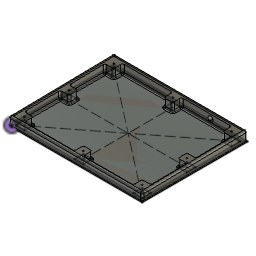
case (Autodesk Fusion 360 design; units mm, degrees)
Autodesk Fusion 360 part; units mm, degrees
sketch "Sketch1" plane through (0, 0, 0) normal (0, 0, 1) x (1, 0, 0)
  line L0 (0, 0) -> (294.692, 0)
  line L1 (294.692, 0) -> (294.692, 230.4)
  line L2 (294.692, 230.4) -> (0, 230.4)
  line L3 (0, 230.4) -> (0, 0)
  line L4 (-4, 234.4) -> (298.692, 234.4)
  line L5 (298.692, 234.4) -> (298.692, -4)
  line L6 (298.692, -4) -> (-4, -4)
  line L7 (-4, -4) -> (-4, 234.4)
  line L8 (4, 226.4) -> (290.692, 226.4)
  line L9 (290.692, 226.4) -> (290.692, 4)
  line L10 (290.692, 4) -> (4, 4)
  line L11 (4, 4) -> (4, 226.4)
  line L12 (4, 226.4) -> (24, 226.4)
  line L13 (24, 226.4) -> (24, 206.4)
  line L14 (24, 206.4) -> (4, 206.4)
  line L15 (4, 206.4) -> (4, 226.4)
  line L16 (4, 4) -> (24, 4)
  line L17 (24, 4) -> (24, 24)
  line L18 (24, 24) -> (4, 24)
  line L19 (4, 24) -> (4, 4)
  line L20 (290.692, 226.4) -> (270.692, 226.4)
  line L21 (270.692, 226.4) -> (270.692, 206.4)
  line L22 (270.692, 206.4) -> (290.692, 206.4)
  line L23 (290.692, 206.4) -> (290.692, 226.4)
  line L24 (290.692, 4) -> (270.692, 4)
  line L25 (270.692, 4) -> (270.692, 24)
  line L26 (270.692, 24) -> (290.692, 24)
  line L27 (290.692, 24) -> (290.692, 4)
  line L28 (4, 4) -> (290.692, 226.4) construction
  line L29 (4, 226.4) -> (290.692, 4) construction
  line L30 (147.346, 4) -> (147.346, 226.4) construction
  line L31 (290.692, 115.2) -> (4, 115.2) construction
  line L32 (137.346, 226.4) -> (157.346, 226.4)
  line L33 (157.346, 226.4) -> (157.346, 206.4)
  line L34 (157.346, 206.4) -> (137.346, 206.4)
  line L35 (137.346, 206.4) -> (137.346, 226.4)
  line L36 (137.346, 4) -> (157.346, 4)
  line L37 (157.346, 4) -> (157.346, 24)
  line L38 (157.346, 24) -> (137.346, 24)
  line L39 (137.346, 24) -> (137.346, 4)
  line L40 (4, 125.2) -> (24, 125.2)
  line L41 (24, 125.2) -> (24, 105.2)
  line L42 (24, 105.2) -> (4, 105.2)
  line L43 (4, 105.2) -> (4, 125.2)
  line L44 (290.692, 125.2) -> (270.692, 125.2)
  line L45 (270.692, 125.2) -> (270.692, 105.2)
  line L46 (270.692, 105.2) -> (290.692, 105.2)
  line L47 (290.692, 105.2) -> (290.692, 125.2)
  line L48 (4, 206.4) -> (24, 226.4) construction
  line L49 (4, 226.4) -> (24, 206.4) construction
  line L50 (137.346, 226.4) -> (157.346, 206.4) construction
  line L51 (137.346, 206.4) -> (157.346, 226.4) construction
  line L52 (4, 125.2) -> (24, 105.2) construction
  line L53 (4, 105.2) -> (24, 125.2) construction
  line L54 (24, 24) -> (4, 4) construction
  line L55 (4, 24) -> (24, 4) construction
  line L56 (137.346, 24) -> (157.346, 4) construction
  line L57 (137.346, 4) -> (157.346, 24) construction
  line L58 (270.692, 24) -> (290.692, 4) construction
  line L59 (270.692, 4) -> (290.692, 24) construction
  line L60 (270.692, 105.2) -> (290.692, 125.2) construction
  line L61 (270.692, 125.2) -> (290.692, 105.2) construction
  line L62 (270.692, 206.4) -> (290.692, 226.4) construction
  line L63 (270.692, 226.4) -> (290.692, 206.4) construction
  dimension "d1" = 294.692
  dimension "d2" = 230.4
  dimension "d3" = 4
  dimension "d4" = 4
  dimension "d5" = 4
  dimension "d6" = 4
  dimension "d7" = 4
  dimension "d8" = 4
  dimension "d9" = 4
  dimension "d10" = 4
  dimension "d11" = 20
  dimension "d12" = 20
  dimension "d13" = 20
  dimension "d14" = 20
  dimension "d15" = 20
  dimension "d16" = 20
  dimension "d17" = 20
  dimension "d18" = 20
  dimension "d19" = 20
  dimension "d20" = 20
  dimension "d21" = 20
  dimension "d22" = 20
  dimension "d23" = 20
  dimension "d24" = 20
  dimension "d25" = 20
  dimension "d26" = 20
  constraint horizontal L0
  constraint vertical L1
  constraint horizontal L2
  constraint vertical L3
  constraint coincident L0.start L3.end
  constraint horizontal L4
  constraint vertical L5
  constraint horizontal L6
  constraint vertical L7
  constraint horizontal L8
  constraint vertical L9
  constraint horizontal L10
  constraint vertical L11
  constraint horizontal L12
  constraint vertical L13
  constraint horizontal L14
  constraint vertical L15
  constraint horizontal L16
  constraint vertical L17
  constraint horizontal L18
  constraint vertical L19
  constraint horizontal L20
  constraint vertical L21
  constraint horizontal L22
  constraint vertical L23
  constraint horizontal L24
  constraint vertical L25
  constraint horizontal L26
  constraint vertical L27
  constraint midpoint L10 L30.start
  constraint midpoint L8 L30.end
  constraint midpoint L9 L31.start
  constraint midpoint L11 L31.end
  constraint horizontal L32
  constraint vertical L33
  constraint horizontal L34
  constraint vertical L35
  constraint coincident L8 L32.start
  constraint symmetric L30 L33 L35
  constraint horizontal L36
  constraint vertical L37
  constraint horizontal L38
  constraint vertical L39
  constraint coincident L10 L36.start
  constraint symmetric L30 L37 L39
  constraint horizontal L40
  constraint vertical L41
  constraint horizontal L42
  constraint vertical L43
  constraint coincident L11 L40.start
  constraint symmetric L31 L40 L42
  constraint horizontal L44
  constraint vertical L45
  constraint horizontal L46
  constraint vertical L47
  constraint coincident L9 L44.start
  constraint symmetric L31 L44 L46
  measures "d1" distance of L0.start L0.end
  measures "d2" distance of L0.start L2.end
  measures "d3" distance of L3 L7
  measures "d4" distance of L2 L4
  measures "d5" distance of L1 L5
  measures "d6" distance of L0 L6
  measures "d7" distance of L3 L11
  measures "d8" distance of L2 L8
  measures "d9" distance of L0 L10
  measures "d10" distance of L1 L9
  measures "d11" distance of L8.start L12.end
  measures "d12" distance of L8.start L14.end
  measures "d13" distance of L10.end L16.end
  measures "d14" distance of L10.end L18.end
  measures "d15" distance of L8.end L20.end
  measures "d16" distance of L8.end L22.end
  measures "d17" distance of L9.end L24.end
  measures "d18" distance of L9.end L26.end
  measures "d19" distance of L32.start L32.end
  measures "d20" distance of L32.start L34.end
  measures "d21" distance of L36.start L36.end
  measures "d22" distance of L36.start L38.end
  measures "d23" distance of L40.start L40.end
  measures "d24" distance of L40.start L42.end
  measures "d25" distance of L44.start L44.end
  measures "d26" distance of L44.start L46.end
extrude "Extrude1" add sketch "Sketch1" along normal blind 20 contours L0 L1 L2 L3 | L4 L5 L6 L7 | L8 L11 L12 L13 L14 L15 | L8 L32 L33 L34 L35 | L11 L40 L41 L42 L43 | L8 L9 L20 L21 L22 L23 | L10 L11 L16 L17 L18 L19 | L9 L44 L45 L46 L47 | L10 L36 L37 L38 L39 | L9 L10 L24 L25 L26 L27
extrude "Extrude2" add sketch "Sketch1" against normal blind 2 contours L0 L1 L2 L3 | L4 L5 L6 L7 | L8 L11 L12 L13 L14 L15 | L8 L9 L10 L11 L13 L14 L17 L18 L21 L22 L25 L26 L33 L34 L35 L37 L38 L39 L40 L41 L42 L44 L45 L46 | L8 L32 L33 L34 L35 | L11 L40 L41 L42 L43 | L8 L9 L20 L21 L22 L23 | L10 L11 L16 L17 L18 L19 | L9 L44 L45 L46 L47 | L10 L36 L37 L38 L39 | L9 L10 L24 L25 L26 L27
fillet "Fillet1" radius 4 28 edges at (24, 226.4, 10) (24, 206.4, 10) (4, 206.4, 10) (4, 125.2, 10) (24, 125.2, 10) (24, 105.2, 10) (4, 105.2, 10) (4, 24, 10) (24, 24, 10) (24, 4, 10) (137.346, 4, 10) (137.346, 24, 10) (157.346, 24, 10) (157.346, 4, 10) (270.692, 4, 10) (270.692, 24, 10) (290.692, 24, 10) (137.346, 226.4, 10) (137.346, 206.4, 10) (157.346, 206.4, 10) (157.346, 226.4, 10) (270.692, 226.4, 10) (270.692, 206.4, 10) (290.692, 206.4, 10) (290.692, 125.2, 10) (270.692, 125.2, 10) (270.692, 105.2, 10) (290.692, 105.2, 10)
fillet "Fillet2" radius 4 56 edges at (136.1744, 225.2284, 0) (80.673, 226.4, 0) (25.1716, 225.2284, 0) (24, 216.4, 0) (22.8284, 207.5716, 0) (14, 206.4, 0) (5.1716, 205.2284, 0) (4, 165.8, 0) (5.1716, 126.3716, 0) (14, 125.2, 0) (22.8284, 124.0284, 0) (24, 115.2, 0) (22.8284, 106.3716, 0) (14, 105.2, 0) (5.1716, 104.0284, 0) (4, 64.6, 0) (5.1716, 25.1716, 0) (14, 24, 0) (22.8284, 22.8284, 0) (24, 14, 0) (25.1716, 5.1716, 0) (80.673, 4, 0) (136.1744, 5.1716, 0) (137.346, 14, 0) (138.5176, 22.8284, 0) (147.346, 24, 0) (156.1744, 22.8284, 0) (157.346, 14, 0) (158.5176, 5.1716, 0) (214.019, 4, 0) (269.5204, 5.1716, 0) (270.692, 14, 0) (271.8636, 22.8284, 0) (280.692, 24, 0) (289.5204, 25.1716, 0) (290.692, 64.6, 0) (289.5204, 104.0284, 0) (280.692, 105.2, 0) (271.8636, 106.3716, 0) (270.692, 115.2, 0) (271.8636, 124.0284, 0) (280.692, 125.2, 0) (289.5204, 126.3716, 0) (290.692, 165.8, 0) (289.5204, 205.2284, 0) (280.692, 206.4, 0) (271.8636, 207.5716, 0) (270.692, 216.4, 0) (269.5204, 225.2284, 0) (214.019, 226.4, 0) (158.5176, 225.2284, 0) (157.346, 216.4, 0) (156.1744, 207.5716, 0) (147.346, 206.4, 0) (138.5176, 207.5716, 0) (137.346, 216.4, 0)
sketch "Sketch2" plane through (0, 0, 20) normal (0, 0, 1) x (-1, 0, 0)
  arc A0 (-270.692, -109.2) -> (-274.692, -105.2) centre (-274.692, -109.2) ccw
  line L0 (-274.692, -105.2) -> (-286.692, -105.2)
  arc A1 (-290.692, -101.2) -> (-286.692, -105.2) centre (-286.692, -101.2) ccw
  line L1 (-290.692, -101.2) -> (-290.692, -28)
  arc A2 (-286.692, -24) -> (-290.692, -28) centre (-286.692, -28) ccw
  line L2 (-286.692, -24) -> (-274.692, -24)
  arc A3 (-274.692, -24) -> (-270.692, -20) centre (-274.692, -20) ccw
  line L3 (-270.692, -20) -> (-270.692, -8)
  arc A4 (-266.692, -4) -> (-270.692, -8) centre (-266.692, -8) ccw
  line L4 (-266.692, -4) -> (-161.346, -4)
  arc A5 (-157.346, -8) -> (-161.346, -4) centre (-161.346, -8) ccw
  line L5 (-157.346, -8) -> (-157.346, -20)
  arc A6 (-157.346, -20) -> (-153.346, -24) centre (-153.346, -20) ccw
  line L6 (-153.346, -24) -> (-141.346, -24)
  arc A7 (-141.346, -24) -> (-137.346, -20) centre (-141.346, -20) ccw
  line L7 (-137.346, -20) -> (-137.346, -8)
  arc A8 (-133.346, -4) -> (-137.346, -8) centre (-133.346, -8) ccw
  line L8 (-133.346, -4) -> (-28, -4)
  arc A9 (-24, -8) -> (-28, -4) centre (-28, -8) ccw
  line L9 (-24, -8) -> (-24, -20)
  arc A10 (-24, -20) -> (-20, -24) centre (-20, -20) ccw
  line L10 (-20, -24) -> (-8, -24)
  arc A11 (-4, -28) -> (-8, -24) centre (-8, -28) ccw
  line L11 (-4, -28) -> (-4, -101.2)
  arc A12 (-8, -105.2) -> (-4, -101.2) centre (-8, -101.2) ccw
  line L12 (-8, -105.2) -> (-20, -105.2)
  arc A13 (-20, -105.2) -> (-24, -109.2) centre (-20, -109.2) ccw
  line L13 (-24, -109.2) -> (-24, -121.2)
  arc A14 (-24, -121.2) -> (-20, -125.2) centre (-20, -121.2) ccw
  line L14 (-20, -125.2) -> (-8, -125.2)
  arc A15 (-4, -129.2) -> (-8, -125.2) centre (-8, -129.2) ccw
  line L15 (-4, -129.2) -> (-4, -202.4)
  arc A16 (-8, -206.4) -> (-4, -202.4) centre (-8, -202.4) ccw
  line L16 (-8, -206.4) -> (-20, -206.4)
  arc A17 (-20, -206.4) -> (-24, -210.4) centre (-20, -210.4) ccw
  line L17 (-24, -210.4) -> (-24, -222.4)
  arc A18 (-28, -226.4) -> (-24, -222.4) centre (-28, -222.4) ccw
  line L18 (-28, -226.4) -> (-133.346, -226.4)
  arc A19 (-137.346, -222.4) -> (-133.346, -226.4) centre (-133.346, -222.4) ccw
  line L19 (-137.346, -222.4) -> (-137.346, -210.4)
  arc A20 (-137.346, -210.4) -> (-141.346, -206.4) centre (-141.346, -210.4) ccw
  line L20 (-141.346, -206.4) -> (-153.346, -206.4)
  arc A21 (-153.346, -206.4) -> (-157.346, -210.4) centre (-153.346, -210.4) ccw
  line L21 (-157.346, -210.4) -> (-157.346, -222.4)
  arc A22 (-161.346, -226.4) -> (-157.346, -222.4) centre (-161.346, -222.4) ccw
  line L22 (-161.346, -226.4) -> (-266.692, -226.4)
  arc A23 (-270.692, -222.4) -> (-266.692, -226.4) centre (-266.692, -222.4) ccw
  line L23 (-270.692, -222.4) -> (-270.692, -210.4)
  arc A24 (-270.692, -210.4) -> (-274.692, -206.4) centre (-274.692, -210.4) ccw
  line L24 (-274.692, -206.4) -> (-286.692, -206.4)
  arc A25 (-290.692, -202.4) -> (-286.692, -206.4) centre (-286.692, -202.4) ccw
  line L25 (-290.692, -202.4) -> (-290.692, -129.2)
  arc A26 (-286.692, -125.2) -> (-290.692, -129.2) centre (-286.692, -129.2) ccw
  line L26 (-286.692, -125.2) -> (-274.692, -125.2)
  arc A27 (-274.692, -125.2) -> (-270.692, -121.2) centre (-274.692, -121.2) ccw
  line L27 (-270.692, -121.2) -> (-270.692, -109.2)
  line L28 (4, 4) -> (-298.692, 4)
  line L29 (-298.692, 4) -> (-298.692, -234.4)
  line L30 (-298.692, -234.4) -> (4, -234.4)
  line L31 (4, -234.4) -> (4, 4)
  line L32 (0, -230.4) -> (-294.692, -230.4)
  line L33 (-294.692, -230.4) -> (-294.692, 0)
  line L34 (-294.692, 0) -> (0, 0)
  line L35 (0, 0) -> (0, -230.4)
  dimension "d35" = 4
  dimension "d36" = 4
  dimension "d37" = 4
  dimension "d38" = 4
  constraint horizontal L32
  constraint vertical L33
  constraint horizontal L34
  constraint vertical L35
  measures "d35" distance of L31 L35
  measures "d36" distance of L30 L32
  measures "d37" distance of L28 L34
  measures "d38" distance of L29 L33
sketch "Sketch3" plane through (-4, 0, 0) normal (-1, 0, 0) x (0, -1, 0)
  line L0 (4, -2) -> (4, 20)
  line L1 (4, 20) -> (-234.4, 20)
  line L2 (-234.4, 20) -> (-234.4, -2)
  line L3 (-234.4, -2) -> (4, -2)
  line L4 (4, -2) -> (4, 16)
  line L5 (4, 16) -> (-234.4, 20)
  dimension "d39" = 18
  constraint coincident L0.start L3.end
  constraint perpendicular L3 L4
  constraint coincident L1.end L2.start
  measures "d39" distance of L0.start L4.end
extrude "Extrude3" cut sketch "Sketch3" against normal through all contours L0 L1 L5
extrude "Extrude4" add sketch "Sketch2" against normal through all of body 1 contours L28 L29 L30 L31
extrude "Extrude5" add 1 faces at (196.4613, -2.6667, 20) along direction (0, 0, 1) blind 3
sketch "Sketch4" plane through (-4, 0, 0) normal (-1, 0, 0) x (0, -1, 0)
  line L0 (-234.4, 23) -> (-234.4, -2)
  line L1 (-234.4, -2) -> (4, -2)
  line L2 (4, -2) -> (4, 23)
  line L3 (4, 23) -> (-234.4, 23)
  line L4 (4, -2) -> (4, 19)
  line L5 (4, 19) -> (-234.4, 23)
  dimension "d44" = 21
  constraint coincident L1.end L2.start
  constraint perpendicular L1 L4
  constraint coincident L0.start L3.end
  measures "d44" distance of L1.end L4.end
extrude "Extrude6" cut sketch "Sketch4" against normal through all contours L2 L3 L5
sketch "Sketch5" plane through (0, 234.4, 0) normal (0, 1, 0) x (-1, 0, 0)
  line L0 (4, -2) -> (4, 23)
  line L1 (4, 23) -> (-298.692, 23)
  line L2 (-298.692, 23) -> (-298.692, -2)
  line L3 (-298.692, -2) -> (4, -2)
  line L4 (-298.692, -2) -> (4, 23) construction
  line L5 (4, -2) -> (-298.692, 23) construction
  line L6 (-147.346, 23) -> (-147.346, -2) construction
  line L7 (-298.692, -2) -> (-147.346, 23) construction
  line L8 (-147.346, -2) -> (-298.692, 23) construction
  circle A0 centre (-223.019, 10.5) radius 5.6
  line L9 (-225.0975, 15.7) -> (-220.9405, 15.7)
  line L10 (-225.0975, 5.3) -> (-220.9405, 5.3)
  dimension "d46" = 11.2
  dimension "d47" = 10.4
  constraint coincident L2.end L3.start
  constraint coincident L0.end L1.start
  constraint coincident L0.start L3.end
  constraint coincident L1.end L2.start
  constraint midpoint L1 L6.start
  constraint midpoint L3 L6.end
  constraint midpoint L7 A0.centre
  constraint coincident A0 L9.start
  constraint coincident A0 L9.end
  constraint horizontal L9
  constraint coincident A0 L10.start
  constraint coincident A0 L10.end
  constraint horizontal L10
  constraint equal L9 L10
  measures "d46" diameter of A0
  measures "d47" distance of L9 L10
extrude "Extrude7" cut sketch "Sketch5" against normal blind 8 contours A0 L9 L10
fillet "Fillet3" radius 2 4 edges at (0, 230.4, 21.4329) (0, 0, 17.5671) (294.692, 0, 17.5671) (294.692, 230.4, 21.4329)
fillet "Fillet4" radius 4 4 edges at (298.692, -4, 8.5) (298.692, 234.4, 10.5) (-4, -4, 8.5) (-4, 234.4, 10.5)
fillet "Fillet5" radius 4 16 edges at (-2.8284, -2.8284, -2) (-4, 115.2, -2) (-2.8284, 233.2284, -2) (147.346, 234.4, -2) (297.5204, 233.2284, -2) (298.692, 115.2, -2) (297.5204, -2.8284, -2) (147.346, -4, -2) (147.346, 234.4, 23) (297.5204, 233.2284, 22.9803) (298.692, 115.2, 21) (297.5204, -2.8284, 19.0197) (147.346, -4, 19) (-2.8284, -2.8284, 19.0197) (-4, 115.2, 21) (-2.8284, 233.2284, 22.9803)
hole "Hole1" at (14, 216.3986, 19.698) direction (0, 0.016776, -0.999859) diameter 3.332 depth 8 tip angle 118
thread "Thread1" "ISO Metric profile 4.0 M4x0.7 6H" major diameter 4.1095 minor diameter 3.332 pitch 0.7 angle 60 resizes the face on face at (12.6473, 215.4709, 17.0154)
hole "Hole2" at (147.346, 216.3986, 19.698) direction (0, 0.016776, -0.999859) diameter 3.332 depth 10 tip angle 118
thread "Thread2" "ISO Metric profile 4.0 M4x0.7 6H" thread offset 0 thread depth 7.4
hole "Hole3" at (280.692, 216.3986, 19.698) direction (0, 0.016776, -0.999859) diameter 3.332 depth 10 tip angle 118
thread "Thread3" "ISO Metric profile 4.0 M4x0.7 6H" thread offset 0 thread depth 7.4
hole "Hole4" at (280.692, 115.2014, 18) direction (0, 0.016776, -0.999859) diameter 3.332 depth 10 tip angle 118
thread "Thread4" "ISO Metric profile 4.0 M4x0.7 6H" thread offset 0 thread depth 7.4
hole "Hole5" at (280.692, 14.0014, 16.302) direction (0, 0.016776, -0.999859) diameter 3.332 depth 10 tip angle 118
thread "Thread5" "ISO Metric profile 4.0 M4x0.7 6H" thread offset 0 thread depth 7.4
hole "Hole6" at (147.346, 14.0014, 16.302) direction (0, 0.016776, -0.999859) diameter 3.332 depth 10 tip angle 118
thread "Thread6" "ISO Metric profile 4.0 M4x0.7 6H" thread offset 0 thread depth 7.4
hole "Hole7" at (14, 14.0014, 16.302) direction (0, 0.016776, -0.999859) diameter 3.332 depth 10 tip angle 118
thread "Thread7" "ISO Metric profile 4.0 M4x0.7 6H" thread offset 0 thread depth 7.4
hole "Hole8" at (14, 115.2014, 18) direction (0, 0.016776, -0.999859) diameter 3.332 depth 10 tip angle 118
thread "Thread8" "ISO Metric profile 4.0 M4x0.7 6H" thread offset 0 thread depth 7.4
